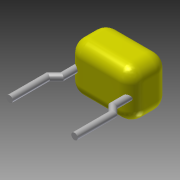
# Autodesk Inventor part: Capacitor
Saved by Autodesk Inventor 2014 SP1 (Build 180222100, 222)
## iProperties
Created: 2016-03-19
Part Number: Capacitor
Material: Generic
Document SubType Name: Modeling
Designer: Tyler
Density: 1 g/cm^3
Appearance: Smooth - Yellow
Author: Tyler
Autodesk Inventor part; units mm, degrees
ref_plane "YZ Plane" through (0, 0, 0) normal (1, 0, 0) x (0, 1, 0)
ref_plane "XZ Plane" through (0, 0, 0) normal (0, 1, 0) x (-1, 0, 0)
ref_plane "XY Plane" through (0, 0, 0) normal (0, 0, 1) x (1, 0, 0)
sketch "Sketch1" plane through (0, 0, 0) normal (0, 0, 1) x (1, 0, 0)
  line L0 (-2.5, -0.5) -> (2.5, -0.5)
  line L1 (2.5, -0.5) -> (2.5, 2.5)
  line L2 (2.5, 2.5) -> (-2.5, 2.5)
  line L3 (-2.5, 2.5) -> (-2.5, -0.5)
  line L4 (-2.5, -0.5) -> (2.5, 2.5) construction
  line L5 (2.5, -0.5) -> (-2.5, 2.5) construction
  point P0 (0, 0)
  point P1 (0, 1)
  dimension "d0" = 5
  dimension "d1" = 3
  dimension "d10" = 1
  dimension "d11" = 0
  constraints: 12 end point, 2 midpoint, 2 parallel, 1 horizontal, 1 perpendicular
  measures "d0" distance of L1.end L2.end
  measures "d1" distance of L0.end L1.end
  measures "d10" distance of point (0, 0) point (0, 1)
  measures "d11" horizontal distance of point (0, 0) point (0, 1)
extrude "Extrusion1" add sketch "Sketch1" along normal mid plane 3.8
sketch "Sketch2" plane through (0, 0, 0) normal (0, 0, 1) x (1, 0, 0)
  line L0 (0, 0) -> (-2, 0)
  line L1 (-2, 0) -> (-2, -1.46)
  line L2 (-2, -1.46) -> (-2.54, -2)
  line L3 (-2.54, -2) -> (-2.54, -5)
  line L4 (0, 0) -> (0, -4.5028) construction
  line L5 (0, 0) -> (2, 0)
  line L6 (2, 0) -> (2, -1.46)
  line L7 (2, -1.46) -> (2.54, -2)
  line L8 (2.54, -2) -> (2.54, -5)
  dimension "d4" = 3
  dimension "d5" = 2.54
  dimension "d6" = 45
  dimension "d8" = 2
  dimension "d9" = 2
  constraints: 18 end point, 4 symmetric about line, 2 parallel, 1 horizontal, 1 perpendicular
  measures "d4" distance of L2.end L3.end
  measures "d5" distance from line of L0.start L3
  measures "d6" angle of L3 L2
  measures "d8" distance from line of L0 L2.end
  measures "d9" distance from line of L0.start L1
fillet "Fillet1" radius 1 12 edges at (0, -0.5, -1.9) (-2.5, 1, -1.9) (0, 2.5, -1.9) (2.5, 1, -1.9) (-2.5, -0.5, 0) (-2.5, 1, 1.9) (-2.5, 2.5, 0) (0, 2.5, 1.9) (2.5, 2.5, 0) (2.5, 1, 1.9) (2.5, -0.5, 0) (0, -0.5, 1.9)
sketch "Sketch3" plane through (0, 0, 0) normal (1, 0, 0) x (0, 1, 0)
  circle A0 centre (0, 0) radius 0.25
  dimension "d13" = 0.5
  constraints: 1 centre point, 1 coincident
  measures "d13" diameter of A0
sweep "Sweep1" add profiles "Sketch3" path "Sketch2"
body "Solid1"
